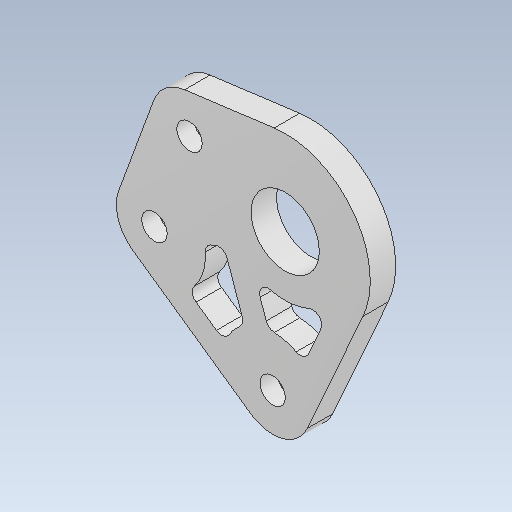
# Autodesk Inventor part: アーム揺動節抑え
Saved by Autodesk Inventor 2020.2 (Build 242310000, 310)
## iProperties
Created: 2020-03-24
Part Number: アーム揺動節抑え
Material: アルミニウム 2014-T4
Document SubType Name: Modeling
Designer: aoyam
Density: 2.8 g/cm^3
Appearance: サテン
Mass: 4.33919 g
Surface Area: 16.8328 cm^2
Volume: 1.54971 cm^3
Author: aoyam
Autodesk Inventor part; units mm, degrees
ref_plane "YZ Plane" through (0, 0, 0) normal (1, 0, 0) x (0, 1, 0)
ref_plane "XZ Plane" through (0, 0, 0) normal (0, 1, 0) x (-1, 0, 0)
ref_plane "XY Plane" through (0, 0, 0) normal (0, 0, 1) x (1, 0, 0)
sketch "スケッチ1" plane through (0, 0, 0) normal (0, 0, 1) x (1, 0, 0)
  circle A0 centre (0, 0) radius 4.025
  line L0 (0, 0) -> (0, -4.025)
  line L1 (0, 0) -> (-1.4816, -16.9353)
  circle A1 centre (-1.4816, -16.9353) radius 1.5
  line L2 (0, 0) -> (-15.4072, -7.1845)
  circle A2 centre (-15.4072, -7.1845) radius 1.5
  line L3 (0, 0) -> (-11.2763, 4.1042)
  circle A3 centre (-11.2763, 4.1042) radius 1.5
  circle A4 centre (0, 0) radius 7.025
  circle A5 centre (0, 0) radius 10.025
  circle A6 centre (-11.2763, 4.1042) radius 4.5
  circle A7 centre (-15.4072, -7.1845) radius 4.5
  circle A8 centre (-1.4816, -16.9353) radius 4.5
  line L4 (-15.5023, 5.6507) -> (-19.6332, -5.6381)
  line L5 (-17.9883, -10.8707) -> (-4.0627, -20.6215)
  line L6 (2.6304, -18.7632) -> (9.1607, -4.072)
  line L7 (-1.2936, 9.9412) -> (-12.3185, 8.5066)
  point P0 (-11.857, 8.5666)
  dimension "d0" = 8.05
  dimension "d1" = 5
  dimension "d2" = 17
  dimension "d3" = 3
  dimension "d4" = 17
  dimension "d5" = 3
  dimension "d6" = 60
  dimension "d7" = 12
  dimension "d8" = 3
  dimension "d9" = 45
  dimension "d12" = 3
  dimension "d18" = 3
  dimension "d19" = 3
  dimension "d20" = 3
  dimension "d21" = 3
  constraints: 16 end point, 7 centre point, 6 point on circle, 6 tangent, 4 coincident, 1 vertical, 1 vertical alignment, 7 other
  measures "d1" angle of L0 L1
  measures "d2" distance of L0.start L1.end
  measures "d3" diameter of A1
  measures "d4" distance of L0.start L2.end
  measures "d5" diameter of A2
  measures "d6" angle of L1 L2
  measures "d7" distance of L0.start L3.end
  measures "d8" diameter of A3
  measures "d9" angle of L2 L3
  measures "d18" radial gap between concentric circles of A4 A5
  measures "d19" diameter of A3
  measures "d20" radial gap between concentric circles of A2 A7
  measures "d21" radial gap between concentric circles of A1 A8
extrude "押し出し1" add sketch "スケッチ1" along normal blind 3 contours A0 L3 A4 L1 | L1 A4 L2 A0 | A0 L2 A4 L3 | A4 L3 A6 A5 L1 | L1 A5 L2 A4 | A4 L2 A5 A6 L3 | A5 L6 A8 L1 | L1 A8 L5 A7 L2 A5 | A6 A5 L3 | L3 A5 A6 | L2 A7 L4 A6 A5 | A8 | A5 A6 | A7 | A6 L7 A5
sketch "スケッチ2" plane through (0, 0, 0) normal (0, 0, -1) x (-1, 0, 0)
  circle A0 centre (11.2763, 4.1042) radius 1.5 projected
  circle A1 centre (15.4072, -7.1845) radius 1.5 projected
  circle A2 centre (1.4816, -16.9353) radius 1.5 projected
  circle A3 centre (11.2763, 4.1042) radius 3
  circle A4 centre (15.4072, -7.1845) radius 3
  circle A5 centre (1.4816, -16.9353) radius 3
  point P0 (0, 0)
  dimension "d13" = 6
  dimension "d14" = 6
  dimension "d15" = 6
  constraints: 3 centre point, 3 coincident
  measures "d13" diameter of A3
  measures "d14" diameter of A4
  measures "d15" diameter of A5
extrude "押し出し2" cut sketch "スケッチ2" against normal blind 1
sketch "スケッチ3" plane through (0, 0, 0) normal (0, 0, -1) x (-1, 0, 0)
  circle A0 centre (11.2763, 4.1042) radius 3 projected
  circle A1 centre (15.4072, -7.1845) radius 3 projected
  circle A2 centre (1.4816, -16.9353) radius 3 projected
  circle A3 centre (0, 0) radius 4.025 projected
  arc A4 (17.9883, -10.8707) -> (19.6332, -5.6381) centre (15.4072, -7.1845) ccw projected
  line L0 (15.5023, 5.6507) -> (19.6332, -5.6381) projected
  arc A5 (15.5023, 5.6507) -> (11.857, 8.5666) centre (11.2763, 4.1042) ccw projected
  line L1 (1.2936, 9.9412) -> (11.857, 8.5666) projected
  arc A6 (1.2936, 9.9412) -> (-9.1607, -4.072) centre (0, 0) ccw projected
  line L2 (-2.6304, -18.7632) -> (-9.1607, -4.072) projected
  arc A7 (-2.6304, -18.7632) -> (4.0627, -20.6215) centre (1.4816, -16.9353) ccw projected
  line L3 (17.9883, -10.8707) -> (4.0627, -20.6215) projected
  arc A8 (0.9065, 6.9663) -> (-6.4194, -2.8535) centre (0, 0) ccw
  line L4 (0.9065, 6.9663) -> (11.4699, 5.5917)
  arc A9 (12.685, 4.6197) -> (11.4699, 5.5917) centre (11.2763, 4.1042) ccw
  line L5 (12.685, 4.6197) -> (16.8159, -6.669)
  arc A10 (16.2676, -8.4132) -> (16.8159, -6.669) centre (15.4072, -7.1845) ccw
  line L6 (16.2676, -8.4132) -> (2.342, -18.164)
  arc A11 (0.111, -17.5446) -> (2.342, -18.164) centre (1.4816, -16.9353) ccw
  line L7 (0.111, -17.5446) -> (-6.4194, -2.8535)
  circle A12 centre (0, 0) radius 7.025
  circle A13 centre (1.4816, -16.9353) radius 6
  circle A14 centre (15.4072, -7.1845) radius 6
  circle A15 centre (11.2763, 4.1042) radius 6
  line L8 (0, 0) -> (15.4072, -7.1845) construction
  line L9 (-0.6339, -1.3595) -> (14.7733, -8.544)
  line L10 (16.0412, -5.825) -> (0.6339, 1.3595)
  arc A16 (0.6339, 1.3595) -> (-0.6339, -1.3595) centre (0, 0) ccw
  arc A17 (14.7733, -8.544) -> (16.0412, -5.825) centre (15.4072, -7.1845) ccw
  line L11 (1.4816, -16.9353) -> (6.3668, -2.9689) construction
  line L12 (2.8975, -17.4306) -> (7.7827, -3.4641)
  line L13 (4.9509, -2.4736) -> (0.0658, -16.4401)
  arc A18 (0.0658, -16.4401) -> (2.8975, -17.4306) centre (1.4816, -16.9353) ccw
  arc A19 (7.7827, -3.4641) -> (4.9509, -2.4736) centre (6.3668, -2.9689) ccw
  point P0 (7.7036, -3.5923)
  point P1 (3.9242, -9.9521)
  point P2 (7.2354, -5.029)
  point P3 (4.8156, -11.9469)
  point P4 (7.1009, -14.8319)
  point P5 (11.5088, -11.7454)
  point P6 (9.5081, -6.0888)
  point P7 (1.9838, -10.9564)
  point P8 (3.735, -5.9498)
  point P9 (-6.4194, -2.8535)
  point P10 (-2.2488, -12.236)
  dimension "d22" = 3
  dimension "d23" = 3
  dimension "d24" = 3
  dimension "d25" = 3
  dimension "d26" = 3
  dimension "d27" = 3
  dimension "d28" = 3
  constraints: 24 end point, 16 point on circle, 11 centre point, 8 tangent, 2 midpoint, 2 parallel, 1 point on line, 10 other
  measures "d22" radial gap between concentric circles of A6 A8
  measures "d24" radial gap between concentric circles of A2 A13
  measures "d25" radial gap between concentric circles of A1 A14
  measures "d26" radial gap between concentric circles of A0 A15
  measures "d27" diameter of A17
  measures "d28" diameter of A19
extrude "押し出し3" cut sketch "スケッチ3" against normal blind 10 contours A12 L13 A13 L7 | A14 L6 A13 L12 L9
fillet "フィレット1" radius 1.05 9 edges at (-1.9838, -10.9564, 1.5) (6.4194, -2.8535, 1.5) (2.2488, -12.236, 1.5) (-3.735, -5.9498, 1.5) (-9.5081, -6.0888, 1.5) (-7.2354, -5.029, 1.5) (-4.8156, -11.9469, 1.5) (-7.1009, -14.8319, 1.5) (-11.5088, -11.7454, 1.5)
